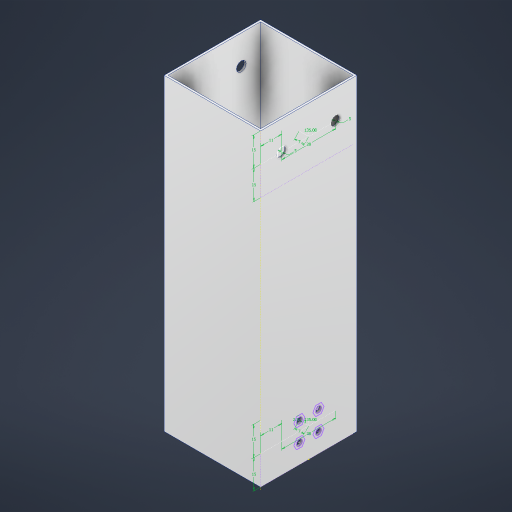
# Autodesk Inventor part: End-Link
Saved by Autodesk Inventor 2023 (Build 270158000, 158)
## iProperties
Created: 2023-08-12
Part Number: End-Link
Material: Aluminum 6061
Document SubType Name: Modeling
Designer: Abhinav
Density: 2.7 g/cm^3
Appearance: Aluminum - Flat
Mass: 84.3073 g
Surface Area: 629.801 cm^2
Volume: 31.2249 cm^3
Author: Abhinav
Autodesk Inventor part; units mm, degrees
ref_plane "YZ Plane" through (0, 0, 0) normal (1, 0, 0) x (0, 1, 0)
ref_plane "XZ Plane" through (0, 0, 0) normal (0, 1, 0) x (-1, 0, 0)
ref_plane "XY Plane" through (0, 0, 0) normal (0, 0, 1) x (1, 0, 0)
sketch "Sketch1" plane through (0, 0, 0) normal (0, 1, 0) x (-1, 0, 0)
  line L0 (25, 25) -> (-25, 25)
  line L1 (-25, 25) -> (-25, -25)
  line L2 (-25, -25) -> (25, -25)
  line L3 (25, -25) -> (25, 25)
  line L4 (25, 25) -> (-25, -25) construction
  line L5 (-25, 25) -> (25, -25) construction
  line L6 (24, 24) -> (-24, 24)
  line L7 (-24, 24) -> (-24, -24)
  line L8 (-24, -24) -> (24, -24)
  line L9 (24, -24) -> (24, 24)
  line L10 (24, 24) -> (-24, -24) construction
  line L11 (-24, 24) -> (24, -24) construction
  point P0 (0, 0)
  dimension "d0" = 50
  dimension "d2" = 48
  constraints: 24 end point, 4 midpoint, 4 parallel, 4 perpendicular, 2 horizontal
  measures "d0" distance of L2.end L1.end
  measures "d2" distance of L8.end L7.end
extrude "Extrusion1" add sketch "Sketch1" along normal blind 160
sketch "Sketch2" plane through (25, 0, 25) normal (1, 0, 0) x (0, 0, -1)
  line L0 (0, 0) -> (48, 0) construction
  line L1 (0, 0) -> (0, 15) construction
  line L2 (0, 15) -> (11, 15) construction
  line L3 (11, 15) -> (39, 15) construction
  line L4 (25, 15) -> (20.0503, 19.9497) construction
  line L5 (25, 15) -> (32, 15) construction
  line L6 (20.0503, 19.9497) -> (20.0503, 22.4497) construction
  line L7 (21.4936, 22.4497) -> (22.937, 19.9497)
  line L8 (22.937, 19.9497) -> (21.4936, 17.4497)
  line L9 (21.4936, 17.4497) -> (18.6069, 17.4497)
  line L10 (18.6069, 17.4497) -> (17.1635, 19.9497)
  line L11 (17.1635, 19.9497) -> (18.6069, 22.4497)
  line L12 (18.6069, 22.4497) -> (21.4936, 22.4497)
  line L13 (25, 15) -> (25, 18.7194) construction
  circle A0 centre (20.0503, 19.9497) radius 1.5
  line L14 (29.9497, 19.9497) -> (29.9497, 22.4497) construction
  line L15 (28.5064, 22.4497) -> (27.063, 19.9497)
  line L16 (27.063, 19.9497) -> (28.5064, 17.4497)
  line L17 (28.5064, 17.4497) -> (31.3931, 17.4497)
  line L18 (31.3931, 22.4497) -> (28.5064, 22.4497)
  line L19 (32.8365, 19.9497) -> (31.3931, 22.4497)
  line L20 (31.3931, 17.4497) -> (32.8365, 19.9497)
  circle A1 centre (29.9497, 19.9497) radius 1.5
  line L21 (20.0503, 10.0503) -> (20.0503, 7.5503) construction
  line L22 (21.4936, 7.5503) -> (22.937, 10.0503)
  line L23 (22.937, 10.0503) -> (21.4936, 12.5503)
  line L24 (21.4936, 12.5503) -> (18.6069, 12.5503)
  line L25 (18.6069, 7.5503) -> (21.4936, 7.5503)
  line L26 (17.1635, 10.0503) -> (18.6069, 7.5503)
  line L27 (18.6069, 12.5503) -> (17.1635, 10.0503)
  circle A2 centre (20.0503, 10.0503) radius 1.5
  line L28 (27.063, 10.0503) -> (28.5064, 12.5503)
  line L29 (28.5064, 12.5503) -> (31.3931, 12.5503)
  line L30 (28.5064, 7.5503) -> (27.063, 10.0503)
  circle A3 centre (29.9497, 10.0503) radius 1.5
  line L31 (31.3931, 12.5503) -> (32.8365, 10.0503)
  line L32 (31.3931, 7.5503) -> (28.5064, 7.5503)
  line L33 (32.8365, 10.0503) -> (31.3931, 7.5503)
  line L34 (29.9497, 10.0503) -> (29.9497, 7.5503) construction
  line L35 (0, 15) -> (0, 30) construction
  line L36 (0, 0) -> (0, 160) construction
  line L37 (25, 145) -> (32, 145) construction
  circle A4 centre (39, 145) radius 2.5
  line L38 (11, 145) -> (39, 145) construction
  line L39 (0, 130) -> (48, 130) construction
  line L40 (25, 145) -> (20.0503, 149.9497) construction
  line L41 (25, 145) -> (25, 148.7194) construction
  line L42 (0, 130) -> (0, 145) construction
  line L43 (0, 145) -> (11, 145) construction
  circle A5 centre (11, 145) radius 2.5
  line L44 (0, 145) -> (0, 160) construction
  point P0 (25, 0)
  point P1 (25, 11.2806)
  dimension "d6" = 15
  dimension "d7" = 11
  dimension "d8" = 28
  dimension "d11" = 7
  dimension "d12" = 135
  dimension "d13" = 2.5
  dimension "d18" = 3
  dimension "d19" = 15
  dimension "d20" = 15
  dimension "d21" = 11
  dimension "d22" = 28
  dimension "d23" = 5
  dimension "d24" = 5
  dimension "d25" = 7
  dimension "d26" = 135
  dimension "d29" = 15
  constraints: 88 end point, 34 symmetric about line, 10 coincident, 6 centre point, 4 horizontal, 3 midpoint, 3 point on line, 3 vertical, 2 equal length, 18 other
  measures "d6" distance of L0.start L1.end
  measures "d7" distance of L1.end L3.start
  measures "d8" distance of L3.start L3.end
  measures "d11" distance of L5.start L4.end
  measures "d12" angle of L5 L4
  measures "d13" distance of L6.start L6.end
  measures "d18" diameter of A0
  measures "d19" distance of L1.end L35.end
  measures "d20" distance of L42.start L42.end
  measures "d21" distance of L42.end L38.start
  measures "d22" distance of L38.start L38.end
  measures "d23" diameter of A5
  measures "d24" diameter of A4
  measures "d25" distance of L37.start L40.end
  measures "d26" angle of L37 L40
  measures "d29" distance of L42.end L44.end
extrude "Extrusion2" cut sketch "Sketch2" against normal blind 50 contours A0 | A1 | A2 | A3 | A4 | A5
body "Solid1"
